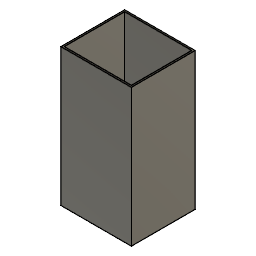
boitier_moteur_roue (Autodesk Fusion 360 design; units mm, degrees)
part number: 2026-05-21-08-46-45-224
Autodesk Fusion 360 part; units mm, degrees
sketch "Esquisse1" plane through (0, 0, 0) normal (0, 0, 1) x (1, 0, 0)
  line L0 (0, 0) -> (21, 0)
  line L1 (21, 0) -> (21, 19)
  line L2 (21, 19) -> (0, 19)
  line L3 (0, 19) -> (0, 0)
  dimension "d1" = 21
  dimension "d2" = 19
  constraint horizontal L0
  constraint vertical L1
  constraint horizontal L2
  constraint vertical L3
  constraint coincident L0.start L3.end
  measures "d1" distance of L0.start L0.end
  measures "d2" distance of L0.start L2.end
extrude "Extrusion1" add sketch "Esquisse1" along normal blind 41
shell "Coque1" thickness 0.5 removed faces 1 at (7, 12.6667, 41)
